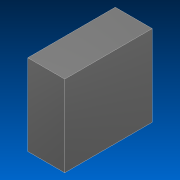
# Autodesk Inventor part: Battery
Saved by Autodesk Inventor 2022.2 (Build 262287000, 287)
## iProperties
Created: 2022-04-13
Part Number: Battery
Material: PET Plastic
Document SubType Name: Modeling
Designer: score_nygvs6w
Density: 1.541 g/cm^3
Appearance: Smooth - Black
Author: score_nygvs6w
Autodesk Inventor part; units mm, degrees
ref_plane "YZ Plane" through (0, 0, 0) normal (1, 0, 0) x (0, 1, 0)
ref_plane "XZ Plane" through (0, 0, 0) normal (0, 1, 0) x (-1, 0, 0)
ref_plane "XY Plane" through (0, 0, 0) normal (0, 0, 1) x (1, 0, 0)
sketch "Sketch1" plane through (0, 0, 0) normal (0, 0, 1) x (1, 0, 0)
  line L0 (-38.1, 83.566) -> (38.1, 83.566)
  line L1 (38.1, 83.566) -> (38.1, -83.566)
  line L2 (38.1, -83.566) -> (-38.1, -83.566)
  line L3 (-38.1, -83.566) -> (-38.1, 83.566)
  line L4 (-38.1, 83.566) -> (38.1, -83.566) construction
  line L5 (38.1, 83.566) -> (-38.1, -83.566) construction
  point P0 (0, 0)
  dimension "d0" = 76.2
  dimension "d1" = 167.132
  constraints: 12 end point, 2 midpoint, 2 parallel, 1 horizontal, 1 perpendicular
  measures "d0" distance of L1.end L2.end
  measures "d1" distance of L0.end L1.end
extrude "Extrusion1" add sketch "Sketch1" along normal mid plane 180.34
body "Solid1"
